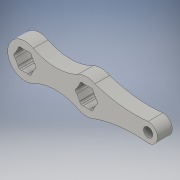
# Autodesk Inventor part: JB_CAD_FinalPt1
Saved by Autodesk Inventor 2016 (Build 200138000, 138)
## iProperties
Created: 2018-06-18
Part Number: JB_CAD_FinalPt1
Material: Generic
Document SubType Name: Modeling
Designer: Student
Density: 1 g/cm^3
Appearance: Default
Author: Student
Autodesk Inventor part; units mm, degrees
ref_plane "YZ Plane" through (0, 0, 0) normal (1, 0, 0) x (0, 1, 0)
ref_plane "XZ Plane" through (0, 0, 0) normal (0, 1, 0) x (-1, 0, 0)
ref_plane "XY Plane" through (0, 0, 0) normal (0, 0, 1) x (1, 0, 0)
sketch "Sketch1" plane through (0, 0, 0) normal (0, 0, 1) x (1, 0, 0)
  line L0 (-11.4295, -0.0912) -> (-11.4381, -0.0912)
  line L1 (-5.798, 9.8601) -> (-5.7937, 9.8528)
  line L2 (5.6401, 9.9513) -> (5.6341, 9.9392)
  line L3 (11.4381, 0.0912) -> (11.4295, 0.0912)
  line L4 (5.798, -9.8601) -> (5.7937, -9.8528)
  line L5 (-5.6401, -9.9513) -> (-5.6341, -9.9392)
  arc A0 (-3.2667, 9.8803) -> (-7.0462, 7.6578) centre (-4.5062, 7.6633) ccw
  arc A1 (7.0443, 7.5633) -> (3.3664, 9.9332) centre (4.5062, 7.6633) ccw
  arc A2 (10.2075, -2.0801) -> (10.1371, 2.3037) centre (8.8895, 0.0912) ccw
  arc A3 (3.2667, -9.8803) -> (7.0462, -7.6578) centre (4.5062, -7.6633) ccw
  arc A4 (-7.0443, -7.5633) -> (-3.3664, -9.9332) centre (-4.5062, -7.6633) ccw
  arc A5 (-10.2075, 2.0801) -> (-10.1371, -2.3037) centre (-8.8895, -0.0912) ccw
  line L6 (-11.4295, -0.1058) -> (-11.4381, -0.0912)
  line L7 (-11.4381, -0.0912) -> (-11.4295, -0.076)
  line L8 (-10.2075, 2.0801) -> (-7.0462, 7.6578)
  line L9 (-5.8064, 9.8453) -> (-5.798, 9.8601)
  line L10 (-5.798, 9.8601) -> (-5.781, 9.8602)
  line L11 (5.6401, 9.9513) -> (5.6527, 9.9298)
  line L12 (-3.2667, 9.8803) -> (3.3664, 9.9332)
  line L13 (5.6098, 9.951) -> (5.6401, 9.9513)
  line L14 (7.0443, 7.5633) -> (10.1371, 2.3037)
  line L15 (11.4295, 0.1058) -> (11.4381, 0.0912)
  line L16 (11.4381, 0.0912) -> (11.4295, 0.076)
  line L17 (10.2075, -2.0801) -> (7.0462, -7.6578)
  line L18 (5.8064, -9.8453) -> (5.798, -9.8601)
  line L19 (5.798, -9.8601) -> (5.781, -9.8602)
  line L20 (-5.6401, -9.9513) -> (-5.6527, -9.9298)
  line L21 (-7.0443, -7.5633) -> (-10.1371, -2.3037)
  line L22 (3.2667, -9.8803) -> (-3.3664, -9.9332)
  line L23 (-5.6098, -9.951) -> (-5.6401, -9.9513)
  arc A6 (8.5907, 15.5669) -> (8.5907, -15.5669) centre (0, 0) ccw
  line L24 (52.0664, -0.0912) -> (52.0579, -0.0912)
  line L25 (57.6979, 9.8601) -> (57.7022, 9.8528)
  line L26 (69.136, 9.9513) -> (69.13, 9.9392)
  line L27 (74.9341, 0.0912) -> (74.9255, 0.0912)
  line L28 (69.294, -9.8601) -> (69.2897, -9.8528)
  line L29 (57.8559, -9.9513) -> (57.8619, -9.9392)
  arc A7 (60.2293, 9.8803) -> (56.4497, 7.6578) centre (58.9897, 7.6633) ccw
  arc A8 (70.5402, 7.5633) -> (66.8624, 9.9332) centre (68.0022, 7.6633) ccw
  arc A9 (73.7034, -2.0801) -> (73.633, 2.3037) centre (72.3855, 0.0912) ccw
  arc A10 (66.7626, -9.8803) -> (70.5422, -7.6578) centre (68.0022, -7.6633) ccw
  arc A11 (56.4517, -7.5633) -> (60.1296, -9.9332) centre (58.9897, -7.6633) ccw
  arc A12 (53.2885, 2.0801) -> (53.3589, -2.3037) centre (54.6064, -0.0912) ccw
  line L30 (52.0665, -0.1058) -> (52.0579, -0.0912)
  line L31 (52.0579, -0.0912) -> (52.0665, -0.076)
  line L32 (53.2885, 2.0801) -> (56.4497, 7.6578)
  line L33 (57.6895, 9.8453) -> (57.6979, 9.8601)
  line L34 (57.6979, 9.8601) -> (57.7149, 9.8602)
  line L35 (69.136, 9.9513) -> (69.1486, 9.9298)
  line L36 (60.2293, 9.8803) -> (66.8624, 9.9332)
  line L37 (69.1057, 9.951) -> (69.136, 9.9513)
  line L38 (70.5402, 7.5633) -> (73.633, 2.3037)
  line L39 (74.9255, 0.1058) -> (74.9341, 0.0912)
  line L40 (74.9341, 0.0912) -> (74.9254, 0.076)
  line L41 (73.7034, -2.0801) -> (70.5422, -7.6578)
  line L42 (69.3024, -9.8453) -> (69.294, -9.8601)
  line L43 (69.294, -9.8601) -> (69.277, -9.8602)
  line L44 (57.8559, -9.9513) -> (57.8433, -9.9298)
  line L45 (56.4517, -7.5633) -> (53.3589, -2.3037)
  line L46 (66.7626, -9.8803) -> (60.1296, -9.9332)
  line L47 (57.8862, -9.951) -> (57.8559, -9.9513)
  circle A13 centre (126.996, -0.1181) radius 4.7625
  arc A14 (124.9667, -9.5543) -> (125.0395, 9.3336) centre (126.996, -0.1181) ccw
  arc A15 (72.0866, 15.5669) -> (126.996, 9.5339) centre (113.0796, 135.7692) ccw
  arc A16 (126.996, -9.7701) -> (72.0866, -15.5669) centre (112.5559, -135.9465) ccw
  arc A17 (54.9053, -15.5669) -> (8.5907, -15.5669) centre (31.748, -60.7817) ccw
  arc A18 (8.5907, 15.5669) -> (54.9053, 15.5669) centre (31.748, 60.7817) ccw
  arc A19 (54.9053, -15.5669) -> (72.0866, -15.5669) centre (63.496, 0) ccw
  arc A20 (72.0866, 15.5669) -> (54.9053, 15.5669) centre (63.496, 0) ccw
  dimension "d19" = 9.525
  dimension "d21" = 19.304
  dimension "d22" = 127
  dimension "d23" = 127
  dimension "d24" = 50.8
  dimension "d25" = 50.8
  constraints: 96 end point, 80 point on circle, 21 centre point, 4 horizontal, 3 coincident, 2 parallel, 14 other
  measures "d19" diameter of A13
  measures "d21" diameter of A14
  measures "d22" radius of A15
  measures "d23" radius of A16
  measures "d24" radius of A17
  measures "d25" radius of A18
extrude "Extrusion1" add sketch "Sketch1" along normal blind 15.24 contours A5 L6 L0 | L0 L7 A5 | L9 L1 A0 | L1 L10 A0 | A3 L4 L19 | A3 L18 L4 | L15 L3 A2 | A2 L3 L16 | A18 A20 A15 A14 A16 A19 A17 A6 | A12 L30 L24 | L24 L31 A12 | L33 L25 A7 | L25 L34 A7 | A10 L28 L43 | A10 L42 L28 | L39 L27 A9 | A9 L27 L40
body "Solid1"
